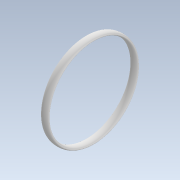
# Autodesk Inventor part: neumatico
Saved by Autodesk Inventor 2021 (Build 250183000, 183)
## iProperties
Created: 2021-04-15
Part Number: neumatico
Material: Genérico
Document SubType Name: Modeling
Designer: j2seb
Density: 1 g/cm^3
Appearance: Valor por defecto
Author: j2seb
Autodesk Inventor part; units mm, degrees
note: some values were not read from the file. Chosen so that the rebuilt part matches the saved one: offset side.
ref_plane "YZ Plane" through (0, 0, 0) normal (1, 0, 0) x (0, 1, 0)
ref_plane "XZ Plane" through (0, 0, 0) normal (0, 1, 0) x (-1, 0, 0)
ref_plane "XY Plane" through (0, 0, 0) normal (0, 0, 1) x (1, 0, 0)
sketch "Boceto1" plane through (0, 0, 0) normal (0, 0, 1) x (1, 0, 0)
  spline S0 degree 5 poles (-24.9404, 274.1789) (-19.9523, 272.5074) (-14.9642, 271.2537) (-9.9761, 270.4179) (0, 269.5821) (9.9761, 270.4179) (14.9642, 271.2537) (19.9523, 272.5074) (24.9404, 274.1789) knots 0 0 0 0 0 0 25.288037 25.288037 25.288037 50.576075 50.576075 50.576075 50.576075 50.576075 50.576075 projected
  line L0 (-27.5011, 282.6709) -> (-27.5011, 0) projected
  line L1 (27.5011, 0) -> (27.5011, 282.6709) projected
  ellipse E0 centre (0, 295) end of major axis (28, 295) minor radius 20
  line L2 (-27.5011, 0) -> (27.5011, 0)
  spline S1 degree 5 poles (25, 295) (25.0002, 296.6194) (24.7089, 298.2423) (24.1276, 299.7855) (22.3467, 302.9903) (19.7286, 305.5804) (18.1158, 306.8169) (14.344, 309.1314) (10.1795, 310.6466) (7.8576, 311.2542) (3.0484, 312.0783) (-1.8315, 312.08) (-4.3082, 311.872) (-8.9625, 311.0727) (-13.3971, 309.4557) (-15.4218, 308.4964) (-18.8869, 306.3826) (-21.7506, 303.5251) (-22.8735, 302.0968) (-24.5346, 299.1286) (-25.1361, 295.7944) (-25.1361, 294.2056) (-24.5346, 290.8714) (-22.8735, 287.9032) (-21.7506, 286.4749) (-18.8869, 283.6174) (-15.4218, 281.5036) (-13.3971, 280.5443) (-8.9625, 278.9273) (-4.3082, 278.128) (-1.8315, 277.92) (3.0484, 277.9217) (7.8576, 278.7458) (10.1795, 279.3534) (14.344, 280.8686) (18.1158, 283.1831) (19.7286, 284.4196) (22.3467, 287.0097) (24.1276, 290.2145) (24.7089, 291.7577) (25.0002, 293.3806) (25, 295) knots 0 0 0 0 0 0 0.060904 0.060904 0.060904 0.136751 0.136751 0.136751 0.226543 0.226543 0.226543 0.319545 0.319545 0.319545 0.403324 0.403324 0.403324 0.470822 0.470822 0.470822 0.529178 0.529178 0.529178 0.596676 0.596676 0.596676 0.680455 0.680455 0.680455 0.773457 0.773457 0.773457 0.863249 0.863249 0.863249 0.939096 0.939096 0.939096 1 1 1 1 1 1
  point P0 (0, 0)
  dimension "d0" = 28
  dimension "d1" = 20
  dimension "d2" = 295
  dimension "d4" = 3
  constraints: 2 end point, 1 centre point, 1 horizontal, 1 vertical alignment, 1 other
  measures "d1" diameter of E0
  measures "d2" distance of point (0, 0) E0.centre
revolve "Revolución1" add sketch "Boceto1" angle 360 about axis through (-27.5011, 0, 0) along (1, 0, 0)
